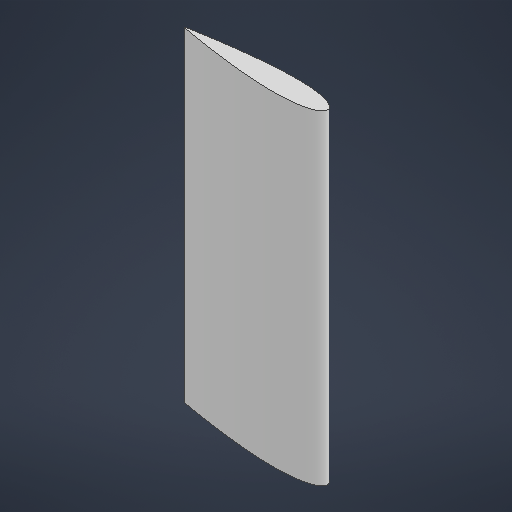
# Autodesk Inventor part: Delb_Tail_v1
Saved by Autodesk Inventor 2026 (Build 300175050, 175E)
## iProperties
Created: 2026-06-09
Part Number: Delb_Tail_v1
Material: Generic
Document SubType Name: Modeling
Designer: Delbe
Density: 1 g/cm^3
Appearance: Default
Author: Delbe
Autodesk Inventor part; units mm, degrees
ref_plane "YZ Plane" through (0, 0, 0) normal (1, 0, 0) x (0, 1, 0)
ref_plane "XZ Plane" through (0, 0, 0) normal (0, 1, 0) x (-1, 0, 0)
ref_plane "XY Plane" through (0, 0, 0) normal (0, 0, 1) x (1, 0, 0)
sketch "Sketch2" plane through (0, 0, 0) normal (0, 1, 0) x (-1, 0, 0)
  spline S0 degree 4 poles (200, 0.3384) (199.9285, 0.3519) (199.5798, 0.4176) (198.995, 0.5274) (198.0088, 0.7116) (196.9736, 0.9037) (195.705, 1.1376) (194.2152, 1.41) (192.5037, 1.7198) (190.5766, 2.0649) (188.4376, 2.4433) (186.0922, 2.8528) (183.5455, 3.2909) (180.8037, 3.7555) (177.8732, 4.2438) (174.7608, 4.7535) (171.4737, 5.2818) (168.0197, 5.8262) (164.4069, 6.384) (160.6436, 6.9526) (156.7387, 7.529) (152.7012, 8.1108) (148.5407, 8.695) (144.2668, 9.2789) (139.8895, 9.8595) (135.4191, 10.4339) (130.8659, 10.9992) (126.2407, 11.5521) (121.5541, 12.0895) (116.8172, 12.6081) (112.041, 13.1046) (107.2368, 13.5756) (102.4155, 14.0177) (97.5886, 14.4272) (92.7674, 14.8008) (87.9629, 15.135) (83.1868, 15.4264) (78.4488, 15.6718) (73.7634, 15.8679) (69.1299, 16.0119) (64.5939, 16.1009) (60.0731, 16.1333) (55.7438, 16.1054) (51.4532, 16.0173) (47.2985, 15.8666) (43.259, 15.6529) (39.3535, 15.3755) (35.5885, 15.0346) (31.9741, 14.6306) (28.5182, 14.1645) (25.2291, 13.6375) (22.1141, 13.0517) (19.1806, 12.4088) (16.4352, 11.7117) (13.8843, 10.9626) (11.5334, 10.1647) (9.3877, 9.3207) (7.4518, 8.4337) (5.7294, 7.5061) (4.2247, 6.5402) (2.9382, 5.5378) (1.878, 4.499) (1.0353, 3.4244) (0.4461, 2.3127) (0.0433, 1.1716) (0.0208, 0.0001) (0.0433, -1.1717) (0.4461, -2.3127) (1.0353, -3.4244) (1.878, -4.499) (2.9382, -5.5378) (4.2247, -6.5402) (5.7294, -7.5061) (7.4518, -8.4337) (9.3877, -9.3207) (11.5334, -10.1647) (13.8843, -10.9626) (16.4352, -11.7117) (19.1806, -12.4088) (22.1141, -13.0517) (25.2291, -13.6375) (28.5182, -14.1645) (31.9741, -14.6306) (35.5885, -15.0346) (39.3535, -15.3755) (43.259, -15.6529) (47.2985, -15.8666) (51.4532, -16.0172) (55.7438, -16.1055) (60.0731, -16.133) (64.5939, -16.101) (69.1299, -16.0119) (73.7634, -15.8679) (78.4488, -15.6717) (83.1868, -15.4264) (87.9629, -15.135) (92.7674, -14.8008) (97.5886, -14.4272) (102.4155, -14.0177) (107.2368, -13.5756) (112.041, -13.1046) (116.8172, -12.6081) (121.5541, -12.0895) (126.2407, -11.5521) (130.8659, -10.9992) (135.4191, -10.4339) (139.8895, -9.8595) (144.2668, -9.2789) (148.5407, -8.695) (152.7012, -8.1108) (156.7387, -7.529) (160.6436, -6.9526) (164.4069, -6.384) (168.0197, -5.8262) (171.4737, -5.2818) (174.7608, -4.7535) (177.8732, -4.2438) (180.8037, -3.7555) (183.5455, -3.2909) (186.0922, -2.8528) (188.4376, -2.4433) (190.5766, -2.0649) (192.5037, -1.7198) (194.2152, -1.41) (195.705, -1.1376) (196.9736, -0.9037) (198.0088, -0.7116) (198.995, -0.5274) (199.5798, -0.4176) (199.9285, -0.3519) (200, -0.3384) knots 0 0 0 0 0 0.00627 0.009959 0.014251 0.019058 0.024323 0.030001 0.036056 0.04246 0.049186 0.056212 0.063517 0.071081 0.078888 0.086921 0.095164 0.103602 0.112222 0.121008 0.129949 0.13903 0.148239 0.157564 0.166991 0.176509 0.186106 0.19577 0.205489 0.215252 0.225046 0.23486 0.244683 0.254503 0.264308 0.274088 0.283831 0.293525 0.30316 0.312732 0.322213 0.331602 0.340885 0.350045 0.359086 0.367989 0.376743 0.385337 0.393758 0.401997 0.41004 0.417877 0.425497 0.432887 0.440037 0.446936 0.453573 0.459942 0.466037 0.471858 0.477412 0.48272 0.487816 0.492755 0.497596 0.502404 0.507245 0.512184 0.51728 0.522588 0.528142 0.533963 0.540058 0.546427 0.553064 0.559963 0.567113 0.574503 0.582123 0.58996 0.598003 0.606242 0.614663 0.623257 0.632011 0.640914 0.649955 0.659115 0.668398 0.677787 0.687268 0.69684 0.706475 0.716169 0.725912 0.735692 0.745497 0.755317 0.76514 0.774954 0.784748 0.794511 0.80423 0.813894 0.823491 0.833009 0.842436 0.851761 0.86097 0.870051 0.878992 0.887778 0.896398 0.904836 0.913079 0.921112 0.928919 0.936483 0.943788 0.950814 0.95754 0.963944 0.969999 0.975677 0.980942 0.985749 0.990041 0.99373 1 1 1 1 1
  line L0 (200, -0.3384) -> (200, 0.3384)
  line L1 (0.0318, 0) -> (60.0318, 0)
  line L2 (60.0318, 0) -> (60.0318, 16.1208)
  line L3 (60.0318, -16.1207) -> (60.0318, 16.1208)
  point P0 (0, 0)
  point P1 (199.8832, 0.3604)
  point P2 (199.5332, 0.4263)
  point P3 (198.9506, 0.5355)
  point P4 (198.137, 0.6875)
  point P5 (197.0942, 0.8811)
  point P6 (195.8246, 1.1152)
  point P7 (194.3312, 1.3883)
  point P8 (192.6175, 1.6986)
  point P9 (190.6874, 2.0443)
  point P10 (188.5456, 2.4232)
  point P11 (186.197, 2.8333)
  point P12 (183.647, 3.2722)
  point P13 (180.9017, 3.7374)
  point P14 (177.9674, 4.2264)
  point P15 (174.8511, 4.7368)
  point P16 (171.5599, 5.2659)
  point P17 (168.1016, 5.8111)
  point P18 (164.4842, 6.3696)
  point P19 (160.7163, 6.9389)
  point P20 (156.8065, 7.5162)
  point P21 (152.764, 8.0987)
  point P22 (148.5983, 8.6837)
  point P23 (144.3192, 9.2683)
  point P24 (139.9365, 9.8496)
  point P25 (135.4605, 10.4246)
  point P26 (130.9017, 10.9904)
  point P27 (126.2707, 11.5438)
  point P28 (121.5784, 12.0817)
  point P29 (116.8357, 12.6007)
  point P30 (112.0537, 13.0974)
  point P31 (107.2435, 13.5686)
  point P32 (102.4164, 14.0107)
  point P33 (97.5836, 14.4202)
  point P34 (92.7565, 14.7937)
  point P35 (87.9463, 15.1276)
  point P36 (83.1643, 15.4185)
  point P37 (78.4216, 15.6633)
  point P38 (73.7293, 15.8587)
  point P39 (69.0983, 16.0018)
  point P40 (64.5395, 16.0899)
  point P41 (55.6808, 16.0919)
  point P42 (51.4017, 16.002)
  point P43 (47.236, 15.8496)
  point P44 (43.1935, 15.6338)
  point P45 (39.2837, 15.3543)
  point P46 (35.5158, 15.0109)
  point P47 (31.8984, 14.6042)
  point P48 (28.4401, 14.1351)
  point P49 (25.1489, 13.6049)
  point P50 (22.0326, 13.0155)
  point P51 (19.0983, 12.3687)
  point P52 (16.353, 11.6672)
  point P53 (13.803, 10.9135)
  point P54 (11.4544, 10.1105)
  point P55 (9.3126, 9.2611)
  point P56 (7.3825, 8.3685)
  point P57 (5.6688, 7.4356)
  point P58 (4.1754, 6.4654)
  point P59 (2.9058, 5.4606)
  point P60 (1.863, 4.424)
  point P61 (1.0494, 3.3578)
  point P62 (0.4668, 2.264)
  point P63 (0.1168, 1.1443)
  point P64 (0.1168, -1.1443)
  point P65 (0.4668, -2.264)
  point P66 (1.0494, -3.3578)
  point P67 (1.863, -4.424)
  point P68 (2.9058, -5.4606)
  point P69 (4.1754, -6.4654)
  point P70 (5.6688, -7.4356)
  point P71 (7.3825, -8.3685)
  point P72 (9.3126, -9.2611)
  point P73 (11.4544, -10.1105)
  point P74 (13.803, -10.9135)
  point P75 (16.353, -11.6672)
  point P76 (19.0983, -12.3687)
  point P77 (22.0326, -13.0155)
  point P78 (25.1489, -13.6049)
  point P79 (28.4401, -14.1351)
  point P80 (31.8984, -14.6042)
  point P81 (35.5158, -15.0109)
  point P82 (39.2837, -15.3543)
  point P83 (43.1935, -15.6338)
  point P84 (47.236, -15.8496)
  point P85 (51.4017, -16.002)
  point P86 (55.6808, -16.0919)
  point P87 (64.5395, -16.0899)
  point P88 (69.0983, -16.0018)
  point P89 (73.7293, -15.8587)
  point P90 (78.4216, -15.6633)
  point P91 (83.1643, -15.4185)
  point P92 (87.9463, -15.1276)
  point P93 (92.7565, -14.7937)
  point P94 (97.5836, -14.4202)
  point P95 (102.4164, -14.0107)
  point P96 (107.2435, -13.5686)
  point P97 (112.0537, -13.0974)
  point P98 (116.8357, -12.6007)
  point P99 (121.5784, -12.0817)
  point P100 (126.2707, -11.5438)
  point P101 (130.9017, -10.9904)
  point P102 (135.4605, -10.4246)
  point P103 (139.9365, -9.8496)
  point P104 (144.3192, -9.2683)
  point P105 (148.5983, -8.6837)
  point P106 (152.764, -8.0987)
  point P107 (156.8065, -7.5162)
  point P108 (160.7163, -6.9389)
  point P109 (164.4842, -6.3696)
  point P110 (168.1016, -5.8111)
  point P111 (171.5599, -5.2659)
  point P112 (174.8511, -4.7368)
  point P113 (177.9674, -4.2264)
  point P114 (180.9017, -3.7374)
  point P115 (183.647, -3.2722)
  point P116 (186.197, -2.8333)
  point P117 (188.5456, -2.4232)
  point P118 (190.6874, -2.0443)
  point P119 (192.6175, -1.6986)
  point P120 (194.3312, -1.3883)
  point P121 (195.8246, -1.1152)
  point P122 (197.0942, -0.8811)
  point P123 (198.137, -0.6875)
  point P124 (198.9506, -0.5355)
  point P125 (199.5332, -0.4263)
  point P126 (199.8832, -0.3604)
  dimension "d6" = 60
  dimension "d7" = 32.2414
  constraints: 8 end point, 1 collinear, 1 horizontal, 1 perpendicular, 1 vertical, 131 other
  measures "d6" distance of L1.start L1.end
  measures "d7" distance of L3.start L2.end
extrude "Extrusion2" add sketch "Sketch2" along normal blind 453.491
body "Solid2"
